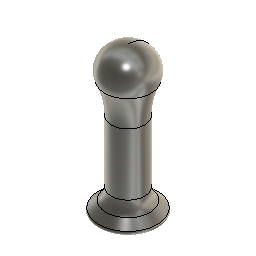
Joystick_ver2_rev_1.1 (Autodesk Fusion 360 design; units mm, degrees)
Autodesk Fusion 360 part; units mm, degrees
sketch "Schizzo1" plane through (0, 0, 0) normal (1, 0, 0) x (0, 1, 0)
  spline S0 degree 4 poles (6.5, 0) (7.1387, -3.4839) (13.3781, -3.3973) (18.2915, -6.9187) (18.8284, -9.0213) knots 0 0 0 0 0 1 1 1 1 1
  line L0 (6.5, 0) -> (7.1387, -3.4839)
  line L1 (7.1387, -3.4839) -> (13.3781, -3.3973)
  line L2 (13.3781, -3.3973) -> (18.2915, -6.9187)
  line L3 (18.2915, -6.9187) -> (18.8284, -9.0213)
  line L4 (3.225, 0) -> (3.225, 15)
  line L5 (15.8979, -3.483) -> (21.2628, -8.3935)
  line L6 (3.225, 0) -> (6.5, 0)
  line L7 (20.25, -9.5) -> (21.75, -9.5) construction
  arc A0 (12.1624, 5) -> (15.8979, -3.483) centre (23.6624, 5) ccw
  line L8 (0, 0) -> (3.225, 0) construction
  line L9 (0, 0) -> (0, 15) construction
  line L10 (3.225, 15) -> (0, 15)
  line L11 (0, 95) -> (0, 15)
  line L12 (20.25, -11) -> (20.25, -9.5) construction
  circle A1 centre (20.25, -9.5) radius 1.5
  line L13 (0, 95) -> (-15, 95) construction
  line L14 (12.1624, 5) -> (12.1624, 50)
  ellipse E0 centre (0, 78.5258) end of major axis (18.2065, 78.5258) minor radius 16.4742 (16.9001, 72.398) -> (0, 95) ccw
  arc A2 (16.9001, 72.398) -> (12.1624, 50) centre (67.476, 50) ccw
  line L15 (0, 81) -> (18, 81) construction
  point P0 (11, 1)
  point P1 (20.25, -11)
  dimension "d1" = 3.225
  dimension "d2" = 15
  dimension "d3" = 6.5
  dimension "d5" = 11
  dimension "d6" = 3
  dimension "d7" = 21.75
  dimension "d8" = 11
  dimension "d9" = 1
  dimension "d17" = 6.24
  dimension "d18" = 3.542
  dimension "d19" = 6.045
  dimension "d20" = 2.17
  dimension "d24" = 11.5
  dimension "d38" = 90
  dimension "d41" = 4
  dimension "d45" = 18
  dimension "d46" = 14
  dimension "d47" = 45
  constraint vertical L4
  constraint perpendicular L4 L10
  constraint coincident L8.start L9.start
  constraint perpendicular L9 L10
  constraint perpendicular L4 L8
  constraint perpendicular L4 L6
  constraint coincident P1 A1
  constraint coincident P1 L12.start
  constraint coincident L7.start L12.end
  constraint vertical L12
  constraint coincident L7.end A1
  constraint perpendicular L7 L12
  constraint coincident S0.end A1
  constraint coincident L5.end A1
  constraint tangent L5 A1
  constraint perpendicular L10 L11
  constraint coincident P0 L5
  constraint tangent L5 A0
  constraint perpendicular L11 L13
  constraint tangent A0 L14
  constraint vertical L14
  constraint tangent E0 A2
  constraint coincident L11 E0.centre
  constraint tangent L13 E0
  constraint tangent L14 A2
  constraint coincident L11 L15.start
  constraint coincident E0 L15.end
  constraint horizontal L15
  measures "d1" distance of L4 L9
  measures "d2" distance of L4.end L4.start
  measures "d3" distance of S0.start L8.start
  measures "d5" distance of P1 L6
  measures "d6" diameter of A1
  measures "d7" distance of L7.end L9
  measures "d8" distance of P0 L9
  measures "d9" distance of P0 S0.start
  measures "d17" distance of L1.end L0.end
  measures "d18" distance of L0.end S0.start
  measures "d19" distance of L1.end L2.end
  measures "d20" distance of S0.end L2.end
  measures "d24" radius of A0
  measures "d38" distance of L13 A0.start
  measures "d41" vertical distance of P0 A0.start
  measures "d45" distance of L15.start L15.end
  measures "d46" distance of L13 L15
  measures "d47" distance of L13 L14.end
revolve "Rivoluzione1" add sketch "Schizzo1" angle 360 about axis through (0, 0, 95) along (0, 0, -1) contours S0 L1 L2 L3 L4 L5 L6 A0 L10 L11 A1 L14 E0 A2 | S0 L1 L2 L3 | A1
chamfer "Smusso1" distance 1 angle 45 1 edges at (-3.0068, 1.1662, 0)
equation "d1 = larghezza_incastro_joystick / 2"
equation "d3 = ( 13 / 2 ) * 1 mm"
equation "d7 = ( 43.5 / 2 ) * 1 mm"
equation "d8 = ( 22 / 2 ) * 1 mm"
equation "altezza_joystick = 90 mm" comment "Modificare questovalore per aumentare o diminuire l'altezza del joystick. (Valore di default 90.00 mm)"
equation "larghezza_incastro_joystick = 6.45 mm" comment "Modificare questo valore per allargare o diminuire il foro dell'incastro del Joystick. (Valore di default 6.45 mm)"
equation "d38 = altezza_joystick"
named bodies: "joystick_2"
